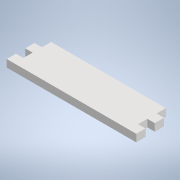
# Autodesk Inventor part: sotto
Saved by Autodesk Inventor 2020.2 (Build 242310000, 310)
## iProperties
Created: 2020-02-13
Part Number: sotto
Material: Generico
Document SubType Name: Modeling
Designer: socci
Density: 1 g/cm^3
Appearance: Default
Author: socci
Autodesk Inventor part; units mm, degrees
ref_plane "YZ Plane" through (0, 0, 0) normal (1, 0, 0) x (0, 1, 0)
ref_plane "XZ Plane" through (0, 0, 0) normal (0, 1, 0) x (-1, 0, 0)
ref_plane "XY Plane" through (0, 0, 0) normal (0, 0, 1) x (1, 0, 0)
sketch "Schizzo1" plane through (0, 0, 0) normal (0, 1, 0) x (-1, 0, 0)
  line L0 (-35, 10) -> (35, 10)
  line L1 (35, 10) -> (35, -10)
  line L2 (35, -10) -> (-35, -10)
  line L3 (-35, -10) -> (-35, 10)
  line L4 (-35, 10) -> (35, -10) construction
  line L5 (35, 10) -> (-35, -10) construction
  point P0 (0, 0)
  dimension "d0" = 70
  dimension "d1" = 20
  constraints: 12 end point, 2 midpoint, 2 parallel, 1 horizontal, 1 perpendicular
  measures "d0" distance of L1.end L2.end
  measures "d1" distance of L0.end L1.end
extrude "Estrusione1" add sketch "Schizzo1" along normal blind 4
sketch "Schizzo2" plane through (0, 0, 0) normal (0, -1, 0) x (1, 0, 0)
  line L0 (-31, 0) -> (-35, 0)
  line L1 (-35, 0) -> (-35, 5)
  line L2 (-35, 5) -> (-31, 5)
  line L3 (-31, 5) -> (-31, 0)
  line L4 (-35, -5) -> (-31, -5)
  line L5 (-31, -5) -> (-31, -10)
  line L6 (-31, -10) -> (-35, -10)
  line L7 (-35, -10) -> (-35, -5)
  line L8 (35, 0) -> (31, 0)
  line L9 (31, 0) -> (31, 5)
  line L10 (31, 5) -> (35, 5)
  line L11 (35, 5) -> (35, 0)
  line L12 (31, -5) -> (35, -5)
  line L13 (35, -5) -> (35, -10)
  line L14 (35, -10) -> (31, -10)
  line L15 (31, -10) -> (31, -5)
  point P0 (0, 0)
  constraints: 32 end point, 8 horizontal, 8 vertical, 16 other
extrude "Estrusione2" cut sketch "Schizzo2" against normal blind 10
